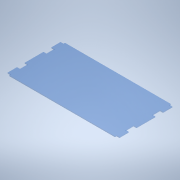
# Autodesk Inventor part: board cover
Saved by Autodesk Inventor 2022 (Build 260153000, 153)
## iProperties
Created: 2021-05-28
Part Number: board cover
Material: Water
Document SubType Name: Modeling
Designer: benka
Density: 0.9983 g/cm^3
Appearance: Tropical Blue
Author: benka
Autodesk Inventor part; units mm, degrees
ref_plane "YZ Plane" through (0, 0, 0) normal (1, 0, 0) x (0, 1, 0)
ref_plane "XZ Plane" through (0, 0, 0) normal (0, 1, 0) x (-1, 0, 0)
ref_plane "XY Plane" through (0, 0, 0) normal (0, 0, 1) x (1, 0, 0)
sketch "Sketch1" plane through (0, 0, 0) normal (0, 1, 0) x (-1, 0, 0)
  line L0 (-94, -88.7502) -> (-94, -93.7502) projected
  line L1 (-104, -88.7502) -> (-94, -88.7502) projected
  line L2 (-104, -57.5002) -> (-104, -88.7502) projected
  line L3 (-94, -57.5002) -> (-104, -57.5002) projected
  line L4 (-94, -31.2502) -> (-94, -57.5002) projected
  line L5 (-104, -31.2502) -> (-94, -31.2502) projected
  line L6 (-104, 31.7498) -> (-104, -31.2502) projected
  line L7 (-94, 31.7498) -> (-104, 31.7498) projected
  line L8 (-94, 57.9998) -> (-94, 31.7498) projected
  line L9 (-104, 57.9998) -> (-94, 57.9998) projected
  line L10 (-104, 89.2498) -> (-104, 57.9998) projected
  line L11 (-94, 89.2498) -> (-104, 89.2498) projected
  line L12 (-94, 94.2498) -> (-94, 89.2498) projected
  line L13 (272, 57.9998) -> (272, 89.2498) projected
  line L14 (262, 57.9998) -> (272, 57.9998) projected
  line L15 (262, 57.9998) -> (262, 31.7498) projected
  line L16 (272, 31.7498) -> (262, 31.7498) projected
  line L17 (262, -31.2502) -> (272, -31.2502) projected
  line L18 (262, -31.2502) -> (262, -57.5002) projected
  line L19 (272, -57.5002) -> (262, -57.5002) projected
  line L20 (272, -88.7502) -> (272, -57.5002) projected
  line L21 (262, -88.7502) -> (272, -88.7502) projected
  line L22 (262, -88.7502) -> (262, -93.7502) projected
  line L23 (262, 89.2498) -> (262, 94.2498)
  line L24 (262, 94.2498) -> (-94, 94.2498) projected
  line L25 (-94, -93.7502) -> (262, -93.7502)
  line L26 (272, 89.2498) -> (262, 89.2498) projected
  line L27 (272, -31.2502) -> (272, 31.7498) projected
  constraints: 4 end point, 1 horizontal, 1 vertical
extrude "Extrusion1" add sketch "Sketch1" along normal blind 3
body "Solid1"
